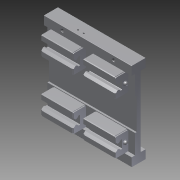
# Autodesk Inventor part: GL15NL-typeExSWNY Table
Saved by Autodesk Inventor 2011 SP1 (Build 150282100, 282)
## iProperties
Created: 2013-10-23
Part Number: GL15NL-typeExSWNY Table
Catalog Web Link: www.cadenas.de
Description: Type GL-N-Y - Table-
Vendor: THK
Document SubType Name: Modeling
Designer: PARTuser1
Manufacturer: THK
Density: 1 g/cm^3
Category: PARTsolutions
Company: THK
Title: GL15NL-typeExSWNY Table
Author: Cadenas PARTsolutions
PSOL_IDENT_0: {$CADENAS_DATA\23d-libs\thk\actuator\type_gl_n\type_gl_n_f_na_s15.prj},206 {VTYP=3D},{NB=GL15NL-type
PSOL_IDENT_1: ExSWNY Table},{LINA=GL15NL-typeExSWNY Table},{NN=Type GL-N-Y - Table},{DATE=01.03.2011 00:58:01},{GE
PSOL_IDENT_2: OMDATE=15.11.2007 14:28:00},{VERSION=},{LINEID=60},{LINESUBID=-1},{WBVAR=S,BSL}  {NB=GL15NL-typeExSW
PSOL_IDENT_3: NY Table},{LINA=GL15NL-typeExSWNY Table},{KT=DUMMY},{IDNR=},{MN=GL15N},{TT=L-type},{TL=154},{B=52},{
PSOL_IDENT_4: C=90},{D=39},{RF=13.250},{RF2=11.550},{L1=53.500},{L2=56.900},{DS=Ex},{S=N},{LM=SW},{BSLX='','None'}
PSOL_IDENT_5: ,{BSL=}
CNS_NB: GL15NL-typeExSWNY Table
CNS_NBSYN: $MN.$TT.$DS.$LM.$S.$BSL.Y Table
CNS_LINA: GL15NL-typeExSWNY Table
CNS_MN: GL15N
CNS_TT: L-type
CNS_TL: 154
CNS_B: 52
CNS_C: 90
CNS_D: 39
CNS_RF: 13.250
CNS_RF2: 11.550
CNS_L1: 53.500
CNS_L2: 56.900
CNS_DS: Ex
CNS_S: N:None
CNS_LM: SW
CNS_BSLX: '','None'
SUPPLIER: THK
ARTICLENO: GL15NL-typeExSWNY Table
BOMINFO: GL15NL-typeExSWNY Table
CREATOR: CADENAS GmbH
Autodesk Inventor part; units mm, degrees
sketch "Sketch_2" plane through (0, 0, 0) normal (1, 0, 0) x (0, 1, 0)
  line L0 (37.6, 77) -> (13.6, 77)
  arc A0 (13.6, 77) -> (13.1, 76.5) centre (13.6, 76.5) ccw
  line L1 (13.1, 76.5) -> (13.1, 62)
  line L2 (13.1, 62) -> (19.1, 62)
  line L3 (19.1, 62) -> (19.1, 28)
  line L4 (19.1, 28) -> (22.1, 28)
  line L5 (22.1, 28) -> (22.1, -28)
  line L6 (22.1, -28) -> (19.1, -28)
  line L7 (19.1, -28) -> (19.1, -62)
  line L8 (19.1, -62) -> (13.1, -62)
  line L9 (13.1, -62) -> (13.1, -76.5)
  arc A1 (13.1, -76.5) -> (13.6, -77) centre (13.6, -76.5) ccw
  line L10 (13.6, -77) -> (37.6, -77)
  line L11 (37.6, -77) -> (37.6, -62)
  line L12 (37.6, -62) -> (30.1, -62)
  arc A2 (29.1, -61) -> (30.1, -62) centre (30.1, -61) ccw
  line L13 (29.1, -61) -> (29.1, 61)
  arc A3 (30.1, 62) -> (29.1, 61) centre (30.1, 61) ccw
  line L14 (30.1, 62) -> (37.6, 62)
  line L15 (37.6, 62) -> (37.6, 77)
  constraints: 32 end point, 8 point on circle, 4 centre point
extrude "Extrusion1" add sketch "Sketch_2" along normal mid plane 154
sketch "Sketch_3" plane through (63.75, 0, 0) normal (1, 0, 0) x (0, 0, -1)
  line L0 (48.7, 18.5) -> (60.25, 18.5)
  line L1 (60.25, 18.5) -> (61.25, 17.5)
  line L2 (61.25, 17.5) -> (61.25, -2.2)
  line L3 (61.25, -2.2) -> (60.25, -3.2)
  line L4 (60.25, -3.2) -> (52.55, -3.2)
  line L5 (52.55, -3.2) -> (53.05, -3.7)
  line L6 (53.05, -3.7) -> (61, -3.7)
  line L7 (61, -3.7) -> (62, -2.7)
  line L8 (62, -2.7) -> (62, 18.1)
  line L9 (62, 18.1) -> (61, 19.1)
  line L10 (61, 19.1) -> (49, 19.1)
  line L11 (49, 19.1) -> (48.7, 18.5)
  constraints: 24 end point
extrude "Extrusion2" add sketch "Sketch_3" against normal blind 53.5
sketch "Sketch_4" plane through (63.75, 0, 0) normal (1, 0, 0) x (0, 0, -1)
  line L0 (28, 18.1) -> (28, -2.7)
  line L1 (28, -2.7) -> (29, -3.7)
  line L2 (29, -3.7) -> (36.95, -3.7)
  line L3 (36.95, -3.7) -> (37.45, -3.2)
  line L4 (37.45, -3.2) -> (29.75, -3.2)
  line L5 (29.75, -3.2) -> (28.75, -2.2)
  line L6 (28.75, -2.2) -> (28.75, 17.5)
  line L7 (28.75, 17.5) -> (29.75, 18.5)
  line L8 (29.75, 18.5) -> (41.3, 18.5)
  line L9 (41.3, 18.5) -> (41, 19.1)
  line L10 (41, 19.1) -> (29, 19.1)
  line L11 (29, 19.1) -> (28, 18.1)
  constraints: 24 end point
extrude "Extrusion3" add sketch "Sketch_4" against normal blind 53.5
sketch "Sketch_5" plane through (65.45, 0, 0) normal (1, 0, 0) x (0, 0, -1)
  line L0 (28.75, 17.6) -> (28.75, -2.2)
  line L1 (28.75, -2.2) -> (29.75, -3.2)
  line L2 (29.75, -3.2) -> (37.45, -3.2)
  line L3 (37.45, -3.2) -> (40.55, -0.1)
  line L4 (40.55, -0.1) -> (40.55, 2.4)
  line L5 (40.55, 2.4) -> (37.45, 5.5)
  line L6 (37.45, 5.5) -> (37.45, 7.37)
  line L7 (37.45, 7.37) -> (38.08, 8)
  line L8 (38.08, 8) -> (51.92, 8)
  line L9 (51.92, 8) -> (52.55, 7.37)
  line L10 (52.55, 7.37) -> (52.55, 5.5)
  line L11 (52.55, 5.5) -> (49.45, 2.4)
  line L12 (49.45, 2.4) -> (49.45, -0.1)
  line L13 (49.45, -0.1) -> (52.55, -3.2)
  line L14 (52.55, -3.2) -> (60.25, -3.2)
  line L15 (60.25, -3.2) -> (61.25, -2.2)
  line L16 (61.25, -2.2) -> (61.25, 17.6)
  line L17 (61.25, 17.6) -> (60.25, 18.6)
  line L18 (60.25, 18.6) -> (29.75, 18.6)
  line L19 (29.75, 18.6) -> (28.75, 17.6)
  constraints: 40 end point
extrude "Extrusion4" add sketch "Sketch_5" against normal blind 56.9
sketch "Sketch_6" plane through (63.75, 0, 0) normal (1, 0, 0) x (0, 0, -1)
  line L0 (-62, 18.1) -> (-62, -2.7)
  line L1 (-62, -2.7) -> (-61, -3.7)
  line L2 (-61, -3.7) -> (-53.05, -3.7)
  line L3 (-53.05, -3.7) -> (-52.55, -3.2)
  line L4 (-52.55, -3.2) -> (-60.25, -3.2)
  line L5 (-60.25, -3.2) -> (-61.25, -2.2)
  line L6 (-61.25, -2.2) -> (-61.25, 17.5)
  line L7 (-61.25, 17.5) -> (-60.25, 18.5)
  line L8 (-60.25, 18.5) -> (-48.7, 18.5)
  line L9 (-48.7, 18.5) -> (-49, 19.1)
  line L10 (-49, 19.1) -> (-61, 19.1)
  line L11 (-61, 19.1) -> (-62, 18.1)
  constraints: 24 end point
extrude "Extrusion5" add sketch "Sketch_6" against normal blind 53.5
sketch "Sketch_7" plane through (63.75, 0, 0) normal (1, 0, 0) x (0, 0, -1)
  line L0 (-41.3, 18.5) -> (-29.75, 18.5)
  line L1 (-29.75, 18.5) -> (-28.75, 17.5)
  line L2 (-28.75, 17.5) -> (-28.75, -2.2)
  line L3 (-28.75, -2.2) -> (-29.75, -3.2)
  line L4 (-29.75, -3.2) -> (-37.45, -3.2)
  line L5 (-37.45, -3.2) -> (-36.95, -3.7)
  line L6 (-36.95, -3.7) -> (-29, -3.7)
  line L7 (-29, -3.7) -> (-28, -2.7)
  line L8 (-28, -2.7) -> (-28, 18.1)
  line L9 (-28, 18.1) -> (-29, 19.1)
  line L10 (-29, 19.1) -> (-41, 19.1)
  line L11 (-41, 19.1) -> (-41.3, 18.5)
  constraints: 24 end point
extrude "Extrusion6" add sketch "Sketch_7" against normal blind 53.5
sketch "Sketch_8" plane through (65.45, 0, 0) normal (1, 0, 0) x (0, 0, -1)
  line L0 (-61.25, 17.6) -> (-61.25, -2.2)
  line L1 (-61.25, -2.2) -> (-60.25, -3.2)
  line L2 (-60.25, -3.2) -> (-52.55, -3.2)
  line L3 (-52.55, -3.2) -> (-49.45, -0.1)
  line L4 (-49.45, -0.1) -> (-49.45, 2.4)
  line L5 (-49.45, 2.4) -> (-52.55, 5.5)
  line L6 (-52.55, 5.5) -> (-52.55, 7.37)
  line L7 (-52.55, 7.37) -> (-51.92, 8)
  line L8 (-51.92, 8) -> (-38.08, 8)
  line L9 (-38.08, 8) -> (-37.45, 7.37)
  line L10 (-37.45, 7.37) -> (-37.45, 5.5)
  line L11 (-37.45, 5.5) -> (-40.55, 2.4)
  line L12 (-40.55, 2.4) -> (-40.55, -0.1)
  line L13 (-40.55, -0.1) -> (-37.45, -3.2)
  line L14 (-37.45, -3.2) -> (-29.75, -3.2)
  line L15 (-29.75, -3.2) -> (-28.75, -2.2)
  line L16 (-28.75, -2.2) -> (-28.75, 17.6)
  line L17 (-28.75, 17.6) -> (-29.75, 18.6)
  line L18 (-29.75, 18.6) -> (-60.25, 18.6)
  line L19 (-60.25, 18.6) -> (-61.25, 17.6)
  constraints: 40 end point
extrude "Extrusion7" add sketch "Sketch_8" against normal blind 56.9
sketch "Sketch_9" plane through (-63.75, 0, 0) normal (1, 0, 0) x (0, 0, -1)
  line L0 (28, 18.1) -> (28, -2.7)
  line L1 (28, -2.7) -> (29, -3.7)
  line L2 (29, -3.7) -> (36.95, -3.7)
  line L3 (36.95, -3.7) -> (37.45, -3.2)
  line L4 (37.45, -3.2) -> (29.75, -3.2)
  line L5 (29.75, -3.2) -> (28.75, -2.2)
  line L6 (28.75, -2.2) -> (28.75, 17.5)
  line L7 (28.75, 17.5) -> (29.75, 18.5)
  line L8 (29.75, 18.5) -> (41.3, 18.5)
  line L9 (41.3, 18.5) -> (41, 19.1)
  line L10 (41, 19.1) -> (29, 19.1)
  line L11 (29, 19.1) -> (28, 18.1)
  constraints: 24 end point
extrude "Extrusion8" add sketch "Sketch_9" along normal blind 53.5
sketch "Sketch_10" plane through (-63.75, 0, 0) normal (1, 0, 0) x (0, 0, -1)
  line L0 (48.7, 18.5) -> (60.25, 18.5)
  line L1 (60.25, 18.5) -> (61.25, 17.5)
  line L2 (61.25, 17.5) -> (61.25, -2.2)
  line L3 (61.25, -2.2) -> (60.25, -3.2)
  line L4 (60.25, -3.2) -> (52.55, -3.2)
  line L5 (52.55, -3.2) -> (53.05, -3.7)
  line L6 (53.05, -3.7) -> (61, -3.7)
  line L7 (61, -3.7) -> (62, -2.7)
  line L8 (62, -2.7) -> (62, 18.1)
  line L9 (62, 18.1) -> (61, 19.1)
  line L10 (61, 19.1) -> (49, 19.1)
  line L11 (49, 19.1) -> (48.7, 18.5)
  constraints: 24 end point
extrude "Extrusion9" add sketch "Sketch_10" along normal blind 53.5
sketch "Sketch_11" plane through (-65.45, 0, 0) normal (1, 0, 0) x (0, 0, -1)
  line L0 (28.75, 17.6) -> (28.75, -2.2)
  line L1 (28.75, -2.2) -> (29.75, -3.2)
  line L2 (29.75, -3.2) -> (37.45, -3.2)
  line L3 (37.45, -3.2) -> (40.55, -0.1)
  line L4 (40.55, -0.1) -> (40.55, 2.4)
  line L5 (40.55, 2.4) -> (37.45, 5.5)
  line L6 (37.45, 5.5) -> (37.45, 7.37)
  line L7 (37.45, 7.37) -> (38.08, 8)
  line L8 (38.08, 8) -> (51.92, 8)
  line L9 (51.92, 8) -> (52.55, 7.37)
  line L10 (52.55, 7.37) -> (52.55, 5.5)
  line L11 (52.55, 5.5) -> (49.45, 2.4)
  line L12 (49.45, 2.4) -> (49.45, -0.1)
  line L13 (49.45, -0.1) -> (52.55, -3.2)
  line L14 (52.55, -3.2) -> (60.25, -3.2)
  line L15 (60.25, -3.2) -> (61.25, -2.2)
  line L16 (61.25, -2.2) -> (61.25, 17.6)
  line L17 (61.25, 17.6) -> (60.25, 18.6)
  line L18 (60.25, 18.6) -> (29.75, 18.6)
  line L19 (29.75, 18.6) -> (28.75, 17.6)
  constraints: 40 end point
extrude "Extrusion10" add sketch "Sketch_11" along normal blind 56.9
sketch "Sketch_12" plane through (-63.75, 0, 0) normal (1, 0, 0) x (0, 0, -1)
  line L0 (-62, 18.1) -> (-62, -2.7)
  line L1 (-62, -2.7) -> (-61, -3.7)
  line L2 (-61, -3.7) -> (-53.05, -3.7)
  line L3 (-53.05, -3.7) -> (-52.55, -3.2)
  line L4 (-52.55, -3.2) -> (-60.25, -3.2)
  line L5 (-60.25, -3.2) -> (-61.25, -2.2)
  line L6 (-61.25, -2.2) -> (-61.25, 17.5)
  line L7 (-61.25, 17.5) -> (-60.25, 18.5)
  line L8 (-60.25, 18.5) -> (-48.7, 18.5)
  line L9 (-48.7, 18.5) -> (-49, 19.1)
  line L10 (-49, 19.1) -> (-61, 19.1)
  line L11 (-61, 19.1) -> (-62, 18.1)
  constraints: 24 end point
extrude "Extrusion11" add sketch "Sketch_12" along normal blind 53.5
sketch "Sketch_13" plane through (-63.75, 0, 0) normal (1, 0, 0) x (0, 0, -1)
  line L0 (-41.3, 18.5) -> (-29.75, 18.5)
  line L1 (-29.75, 18.5) -> (-28.75, 17.5)
  line L2 (-28.75, 17.5) -> (-28.75, -2.2)
  line L3 (-28.75, -2.2) -> (-29.75, -3.2)
  line L4 (-29.75, -3.2) -> (-37.45, -3.2)
  line L5 (-37.45, -3.2) -> (-36.95, -3.7)
  line L6 (-36.95, -3.7) -> (-29, -3.7)
  line L7 (-29, -3.7) -> (-28, -2.7)
  line L8 (-28, -2.7) -> (-28, 18.1)
  line L9 (-28, 18.1) -> (-29, 19.1)
  line L10 (-29, 19.1) -> (-41, 19.1)
  line L11 (-41, 19.1) -> (-41.3, 18.5)
  constraints: 24 end point
extrude "Extrusion12" add sketch "Sketch_13" along normal blind 53.5
sketch "Sketch_14" plane through (-65.45, 0, 0) normal (1, 0, 0) x (0, 0, -1)
  line L0 (-61.25, 17.6) -> (-61.25, -2.2)
  line L1 (-61.25, -2.2) -> (-60.25, -3.2)
  line L2 (-60.25, -3.2) -> (-52.55, -3.2)
  line L3 (-52.55, -3.2) -> (-49.45, -0.1)
  line L4 (-49.45, -0.1) -> (-49.45, 2.4)
  line L5 (-49.45, 2.4) -> (-52.55, 5.5)
  line L6 (-52.55, 5.5) -> (-52.55, 7.37)
  line L7 (-52.55, 7.37) -> (-51.92, 8)
  line L8 (-51.92, 8) -> (-38.08, 8)
  line L9 (-38.08, 8) -> (-37.45, 7.37)
  line L10 (-37.45, 7.37) -> (-37.45, 5.5)
  line L11 (-37.45, 5.5) -> (-40.55, 2.4)
  line L12 (-40.55, 2.4) -> (-40.55, -0.1)
  line L13 (-40.55, -0.1) -> (-37.45, -3.2)
  line L14 (-37.45, -3.2) -> (-29.75, -3.2)
  line L15 (-29.75, -3.2) -> (-28.75, -2.2)
  line L16 (-28.75, -2.2) -> (-28.75, 17.6)
  line L17 (-28.75, 17.6) -> (-29.75, 18.6)
  line L18 (-29.75, 18.6) -> (-60.25, 18.6)
  line L19 (-60.25, 18.6) -> (-61.25, 17.6)
  constraints: 40 end point
extrude "Extrusion13" add sketch "Sketch_14" along normal blind 56.9
sketch "Sketch14" plane through (-77, 13.1, -76.5) normal (0, -1, 0) x (1, 0, 0)
  point P0 (32, 6.5)
hole "Drilling 1" at (-45, 13.1, -70) direction (0, 1, 0) diameter 4.917 depth 24.5 countersink diameter 6 countersink angle 90 thread size "M6x1" class "6H" standard "ISO Metric profile"
sketch "Sketch15" plane through (-77, 13.1, 76.5) normal (0, -1, 0) x (1, 0, 0)
  point P0 (32, -6.5)
hole "Drilling 2" at (-45, 13.1, 70) direction (0, 1, 0) diameter 4.917 depth 24.5 countersink diameter 6 countersink angle 90 thread size "M6x1" class "6H" standard "ISO Metric profile"
sketch "Sketch16" plane through (-77, 13.1, -76.5) normal (0, -1, 0) x (1, 0, 0)
  point P0 (122, 6.5)
hole "Drilling 3" at (45, 13.1, -70) direction (0, 1, 0) diameter 4.917 depth 24.5 countersink diameter 6 countersink angle 90 thread size "M6x1" class "6H" standard "ISO Metric profile"
sketch "Sketch17" plane through (-77, 13.1, 76.5) normal (0, -1, 0) x (1, 0, 0)
  point P0 (122, -6.5)
hole "Drilling 4" at (45, 13.1, 70) direction (0, 1, 0) diameter 4.917 depth 24.5 countersink diameter 6 countersink angle 90 thread size "M6x1" class "6H" standard "ISO Metric profile"
sketch "Sketch_19" plane through (-25, 0, 0) normal (1, 0, 0) x (0, 0, -1)
  line L0 (-71, 21.1) -> (-77, 21.1)
  line L1 (-77, 21.1) -> (-77, 22.6)
  line L2 (-77, 22.6) -> (-76.7295, 22.3295)
  line L3 (-76.7295, 22.3295) -> (-71.2705, 22.3295)
  line L4 (-71.2705, 22.3295) -> (-71, 22.6)
  line L5 (-71, 22.6) -> (-71, 21.1)
  line L6 (-71, 21.1) -> (-77, 21.1)
  constraints: 14 end point
revolve "Revolution1" cut sketch "Sketch_19" angle 360 about axis through (-25, 21.1, 71) along (0, 0, -1)
thread "Thread1" size "M3x0.5" class "6H" standard "ISO Metric profile" full length
sketch "Sketch_20" plane through (-15, 0, 0) normal (1, 0, 0) x (0, 0, -1)
  line L0 (-71, 21.1) -> (-77, 21.1)
  line L1 (-77, 21.1) -> (-77, 22.6)
  line L2 (-77, 22.6) -> (-76.7295, 22.3295)
  line L3 (-76.7295, 22.3295) -> (-71.2705, 22.3295)
  line L4 (-71.2705, 22.3295) -> (-71, 22.6)
  line L5 (-71, 22.6) -> (-71, 21.1)
  line L6 (-71, 21.1) -> (-77, 21.1)
  constraints: 14 end point
revolve "Revolution2" cut sketch "Sketch_20" angle 360 about axis through (-15, 21.1, 71) along (0, 0, -1)
thread "Thread2" size "M3x0.5" class "6H" standard "ISO Metric profile" full length
sketch "Sketch_21" plane through (0, 0, -45) normal (0, 0, 1) x (1, 0, 0)
  line L0 (69.85, 13.1) -> (65.45, 13.1)
  line L1 (65.45, 13.1) -> (65.45, 16.85)
  line L2 (65.45, 16.85) -> (65.85, 16.85)
  line L3 (65.85, 16.85) -> (65.85, 16.1)
  line L4 (65.85, 16.1) -> (66.85, 16.1)
  arc A0 (69.85, 13.1) -> (66.85, 16.1) centre (66.85, 13.1) ccw
  line L5 (69.85, 13.1) -> (65.45, 13.1)
  constraints: 12 end point, 2 point on circle, 1 centre point
revolve "Revolution3" add sketch "Sketch_21" angle 360 about axis through (69.85, 13.1, -45) along (1, 0, 0)
sketch "Sketch_22" plane through (0, 0, -45) normal (0, 0, 1) x (1, 0, 0)
  line L0 (-65.45, 13.1) -> (-69.85, 13.1)
  arc A0 (-66.85, 16.1) -> (-69.85, 13.1) centre (-66.85, 13.1) ccw
  line L1 (-66.85, 16.1) -> (-65.85, 16.1)
  line L2 (-65.85, 16.1) -> (-65.85, 16.85)
  line L3 (-65.85, 16.85) -> (-65.45, 16.85)
  line L4 (-65.45, 16.85) -> (-65.45, 13.1)
  line L5 (-65.45, 13.1) -> (-69.85, 13.1)
  constraints: 12 end point, 2 point on circle, 1 centre point
revolve "Revolution4" add sketch "Sketch_22" angle 360 about axis through (-65.45, 13.1, -45) along (1, 0, 0)
sketch "Sketch_23" plane through (0, 0, 45) normal (0, 0, 1) x (1, 0, 0)
  line L0 (69.85, 13.1) -> (65.45, 13.1)
  line L1 (65.45, 13.1) -> (65.45, 16.85)
  line L2 (65.45, 16.85) -> (65.85, 16.85)
  line L3 (65.85, 16.85) -> (65.85, 16.1)
  line L4 (65.85, 16.1) -> (66.85, 16.1)
  arc A0 (69.85, 13.1) -> (66.85, 16.1) centre (66.85, 13.1) ccw
  line L5 (69.85, 13.1) -> (65.45, 13.1)
  constraints: 12 end point, 2 point on circle, 1 centre point
revolve "Revolution5" add sketch "Sketch_23" angle 360 about axis through (69.85, 13.1, 45) along (1, 0, 0)
sketch "Sketch_24" plane through (0, 0, 45) normal (0, 0, 1) x (1, 0, 0)
  line L0 (-65.45, 13.1) -> (-69.85, 13.1)
  arc A0 (-66.85, 16.1) -> (-69.85, 13.1) centre (-66.85, 13.1) ccw
  line L1 (-66.85, 16.1) -> (-65.85, 16.1)
  line L2 (-65.85, 16.1) -> (-65.85, 16.85)
  line L3 (-65.85, 16.85) -> (-65.45, 16.85)
  line L4 (-65.45, 16.85) -> (-65.45, 13.1)
  line L5 (-65.45, 13.1) -> (-69.85, 13.1)
  constraints: 12 end point, 2 point on circle, 1 centre point
revolve "Revolution6" add sketch "Sketch_24" angle 360 about axis through (-65.45, 13.1, 45) along (1, 0, 0)
ref_plane "type_gl_n_t1_XY" through (-77, 0, 0) normal (1, 0, 0) x (0, 0, -1)
ref_plane "type_gl_n_t1_YZ" through (-77, 0, 0) normal (0, 0, -1) x (0, 1, 0)
ref_plane "type_gl_n_t1_ZX" through (-77, 0, 0) normal (0, 1, 0) x (1, 0, 0)
body "Solid1"
